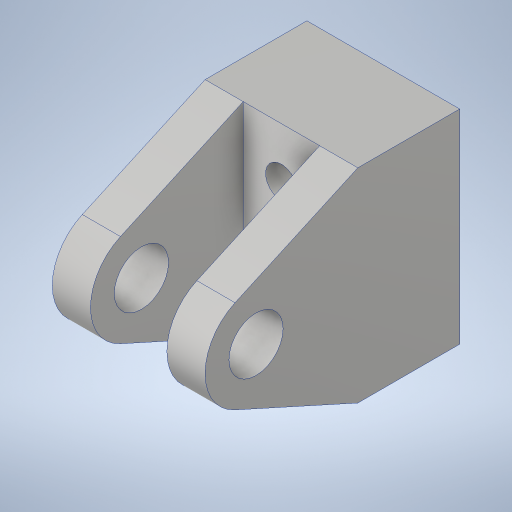
# Autodesk Inventor part: EL2-026-minusfillet
Saved by Autodesk Inventor 2023.4 (Build 274418000, 418)
## iProperties
Created: 2025-02-12
Part Number: EL2-026-minusfillet
Material: Aluminum 6061
Document SubType Name: Modeling
Designer: slick
Density: 2.7 g/cm^3
Appearance: Aluminum - Flat
Author: slick
Autodesk Inventor part; units mm, degrees
ref_plane "YZ Plane" through (0, 0, 0) normal (1, 0, 0) x (0, 1, 0)
ref_plane "XZ Plane" through (0, 0, 0) normal (0, 1, 0) x (-1, 0, 0)
ref_plane "XY Plane" through (0, 0, 0) normal (0, 0, 1) x (1, 0, 0)
sketch "Sketch1" plane through (0, 0, 0) normal (1, 0, 0) x (0, 1, 0)
  line L0 (12.7, 6.35) -> (-12.7, 6.35) construction
  line L1 (-12.7, 6.35) -> (-12.7, -6.35)
  line L2 (-12.7, -6.35) -> (12.7, -6.35)
  line L3 (12.7, -6.35) -> (12.7, 6.35)
  line L4 (12.7, 6.35) -> (-12.7, -6.35) construction
  line L5 (-12.7, 6.35) -> (12.7, -6.35) construction
  circle A0 centre (0, 19.05) radius 6.35 construction
  line L6 (5.7876, 21.6626) -> (12.7, 6.35)
  line L7 (-5.7876, 21.6626) -> (-12.7, 6.35)
  arc A1 (5.7876, 21.6626) -> (-5.7876, 21.6626) centre (0, 19.05) ccw
  point P0 (0, 0)
  point P1 (0, 6.35)
  dimension "d0" = 25.4
  dimension "d1" = 12.7
  dimension "d2" = 12.7
  dimension "d3" = 12.7
  constraints: 16 end point, 5 point on circle, 3 midpoint, 2 centre point, 2 coincident, 2 parallel, 2 tangent, 1 concentric, 1 horizontal, 1 perpendicular, 1 vertical alignment
  measures "d0" distance of L2.end L1.end
  measures "d1" distance of L1.end L0.end
  measures "d2" diameter of A0
  measures "d3" distance of point (0, 6.35) A0.centre
extrude "Extrusion1" add sketch "Sketch1" along normal blind 19.05
hole "Hole1" at (0, 0, 19.05) direction (1, 0, 0) diameter 6.7564 end through all clearance for "Flat Head Machine Screw (82)" size "1/4" standard "Ansi Unified Screw Threads"
sketch "Sketch2" plane through (0, -12.7, -6.35) normal (0, 0, -1) x (-1, 0, 0)
  line L0 (0, 25.4) -> (-19.05, 25.4) construction
  line L1 (0, 0) -> (-19.05, 0) construction
  line L2 (-9.525, 19.05) -> (-9.525, 6.35) construction
  line L3 (0, 0) -> (0, 25.4) construction
  point P0 (0, 12.7)
  point P1 (-9.525, 25.4)
  point P2 (-9.525, 0)
  point P3 (-9.525, 12.7)
  point P4 (0, 12.7)
  dimension "d13" = 12.7
  constraints: 4 midpoint, 3 vertical alignment, 2 end point, 1 horizontal alignment, 1 vertical
  measures "d13" distance of L2.start L2.end
hole "Hole2" at (9.525, 6.35, -6.35) at (9.525, -6.35, -6.35) direction (0, 0, 1) diameter 3.9624 depth 13.6144 tip angle 118 thread size "10-32 UNF" class "2B" standard "ANSI Unified Screw Threads"
sketch "Sketch3" plane through (0, 12.7, 6.35) normal (0, 1, 0) x (1, 0, 0)
  line L0 (0, -15.3126) -> (0, -15.3126) construction
  line L1 (0, -15.3126) -> (19.05, -15.3126) construction
  line L2 (19.05, -15.3126) -> (19.05, -15.3126) construction
  line L3 (0, -15.3126) -> (19.05, -15.3126) construction
  line L4 (0, 0) -> (0, -15.3126) construction
  line L5 (0, -15.3126) -> (19.05, -15.3126) construction
  line L6 (19.05, 0) -> (19.05, -15.3126) construction
  line L7 (0, 0) -> (19.05, 0) construction
  line L8 (0, 12.7) -> (0, 0) construction
  line L9 (0, 0) -> (19.05, 0) construction
  line L10 (19.05, 12.7) -> (19.05, 0) construction
  line L11 (0, 12.7) -> (19.05, 12.7) construction
  line L12 (0, -19.05) -> (19.05, -19.05) construction
  line L13 (4.7625, -19.05) -> (14.2875, -19.05)
  line L14 (14.2875, -19.05) -> (14.2875, 0)
  line L15 (14.2875, 0) -> (4.7625, 0)
  line L16 (4.7625, 0) -> (4.7625, -19.05)
  point P0 (0, 6.35)
  point P1 (9.525, -19.05)
  point P2 (9.525, -19.05)
  dimension "d21" = 9.525
  dimension "d22" = 19.05
  constraints: 8 end point, 2 midpoint, 2 parallel, 1 coincident, 1 horizontal, 1 perpendicular, 1 point on line
  measures "d21" distance between parallel lines of L14 L16
  measures "d22" distance of L15.end L13.start
extrude "Extrusion2" cut sketch "Sketch3" against normal through all
body "Solid1"
